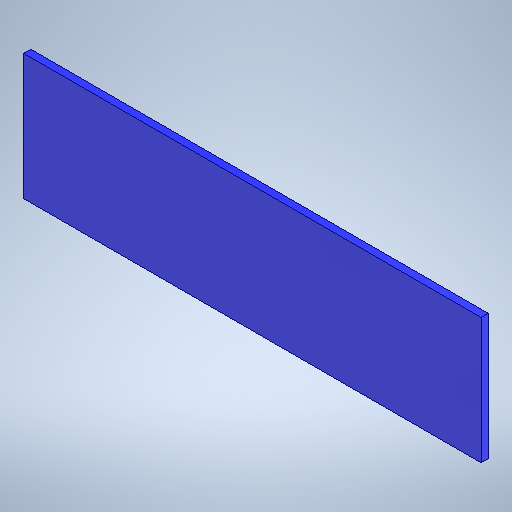
# Autodesk Inventor part: передний кожух
Saved by Autodesk Inventor 2025 (Build 290162000, 162)
## iProperties
Created: 2025-03-01
Part Number: передний кожух
Material: Типовые
Document SubType Name: Modeling
Designer: volko
Density: 1 g/cm^3
Appearance: Синий — малярная краска — глянцевая
Author: volko
Autodesk Inventor part; units mm, degrees
ref_plane "YZ Plane" through (0, 0, 0) normal (1, 0, 0) x (0, 1, 0)
ref_plane "XZ Plane" through (0, 0, 0) normal (0, 1, 0) x (-1, 0, 0)
ref_plane "XY Plane" through (0, 0, 0) normal (0, 0, 1) x (1, 0, 0)
sketch "Эскиз1" plane through (0, 0, 0) normal (0, 0, 1) x (1, 0, 0)
  line L0 (-160, 44) -> (160, 44)
  line L1 (160, 44) -> (160, -44)
  line L2 (160, -44) -> (-160, -44)
  line L3 (-160, -44) -> (-160, 44)
  line L4 (0, -61.6) -> (0, 61.6) projected
  line L5 (-224, 0) -> (224, 0) projected
  point P0 (0, 0)
  dimension "d0" = 88
  dimension "d1" = 320
  constraints: 8 end point, 2 parallel, 1 horizontal, 1 perpendicular, 2 other
  measures "d0" distance of L2.end L0.start
  measures "d1" distance of L0.start L0.end
extrude "Выдавливание1" add sketch "Эскиз1" along normal blind 5
